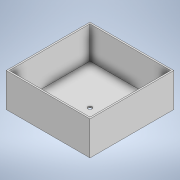
# Autodesk Inventor part: Base
Saved by Autodesk Inventor 2022 (Build 260153000, 153)
## iProperties
Created: 2022-02-27
Part Number: Base
Material: Generic
Document SubType Name: Modeling
Designer: alexo
Density: 1 g/cm^3
Appearance: Default
Author: alexo
Autodesk Inventor part; units mm, degrees
ref_plane "YZ Plane" through (0, 0, 0) normal (1, 0, 0) x (0, 1, 0)
ref_plane "XZ Plane" through (0, 0, 0) normal (0, 1, 0) x (-1, 0, 0)
ref_plane "XY Plane" through (0, 0, 0) normal (0, 0, 1) x (1, 0, 0)
sketch "Sketch1" plane through (0, 0, 0) normal (0, 1, 0) x (-1, 0, 0)
  line L0 (-80.6, -80.6) -> (80.6, -80.6)
  line L1 (80.6, -80.6) -> (80.6, 80.6)
  line L2 (80.6, 80.6) -> (-80.6, 80.6)
  line L3 (-80.6, 80.6) -> (-80.6, -80.6)
  line L4 (-80.6, -80.6) -> (80.6, 80.6) construction
  line L5 (80.6, -80.6) -> (-80.6, 80.6) construction
  point P0 (0, 0)
  dimension "d0" = 161.2
  constraints: 12 end point, 2 midpoint, 2 parallel, 2 perpendicular, 1 horizontal
  measures "d0" distance of L0.end L1.end
extrude "Extrusion1" add sketch "Sketch1" along normal blind 3
sketch "Sketch2" plane through (0, 3, 0) normal (0, 1, 0) x (1, 0, 0)
  line L0 (-80.6, 80.6) -> (-80.6, -80.6) projected
  line L1 (-80.6, -80.6) -> (80.6, -80.6) projected
  line L2 (80.6, -80.6) -> (80.6, 80.6) projected
  line L3 (80.6, 80.6) -> (-80.6, 80.6) projected
  line L4 (77.6, 77.6) -> (-77.6, 77.6)
  line L5 (-77.6, 77.6) -> (-77.6, -77.6)
  line L6 (-77.6, -77.6) -> (77.6, -77.6)
  line L7 (77.6, -77.6) -> (77.6, 77.6)
  line L8 (77.6, 77.6) -> (-77.6, -77.6) construction
  line L9 (-77.6, 77.6) -> (77.6, -77.6) construction
  point P0 (0, 0)
  dimension "d3" = 3
  dimension "d4" = 3
  constraints: 12 end point, 2 midpoint, 2 parallel, 1 horizontal, 1 perpendicular
  measures "d3" distance between parallel lines of L0 L5
  measures "d4" distance between parallel lines of L1 L6
extrude "Extrusion2" add sketch "Sketch2" along normal blind 62
sketch "Sketch3" plane through (0, 3, 0) normal (0, 1, 0) x (1, 0, 0)
  circle A0 centre (0, 0) radius 4
  dimension "d7" = 8
  constraints: 1 centre point, 1 coincident
  measures "d7" diameter of A0
extrude "Extrusion3" cut sketch "Sketch3" against normal blind 44.5
equation "\"d0\" = Lenght"
equation "\"d1\" = Gr"
equation "\"d3\" = Gr"
equation "\"d4\" = Gr"
equation "\"Gr\" = 3"
equation "\"Lenght\" = 161.2"
body "Solid1"
